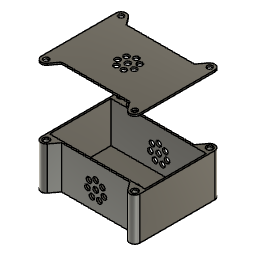
Boitier (Autodesk Fusion 360 design; units mm, degrees)
Autodesk Fusion 360 part; units mm, degrees
sketch "Esquisse2" plane through (0, 0, 0) normal (0, 0, 1) x (1, 0, 0)
  line L0 (29, -22) -> (29, 21.9996)
  line L1 (20, 19) -> (-20, 19)
  line L2 (-29, 21.9997) -> (-29, -21.9996)
  circle A0 centre (-26, -22) radius 1.4
  line L3 (-23.6, -23.8) -> (-20, -19)
  line L4 (-23.6, 23.8) -> (-20, 19)
  line L5 (23.6, -23.8) -> (20, -19)
  line L6 (23.6, 23.8) -> (20, 19)
  line L7 (-26.0004, -19) -> (-25.9996, -19)
  line L8 (-20, -19) -> (20, -19)
  arc A1 (-29, -21.9996) -> (-23.6, -23.8) centre (-26, -22) ccw
  circle A2 centre (-26, 22) radius 1.4
  circle A3 centre (26, 22) radius 1.4
  arc A4 (-23.6, 23.8) -> (-29, 21.9997) centre (-26, 22) ccw
  arc A5 (29, 21.9996) -> (23.6, 23.8) centre (26, 22) ccw
  arc A6 (23.6, -23.8) -> (29, -22) centre (26, -22) ccw
  line L9 (-28, -18) -> (28, -18)
  line L10 (28, -18) -> (28, 18)
  line L11 (28, 18) -> (-28, 18)
  line L12 (-28, 18) -> (-28, -18)
  circle A7 centre (26, -22) radius 1.4
  circle A8 centre (-26, -22) radius 1.55
  circle A9 centre (-26, 22) radius 1.55
  circle A10 centre (26, 22) radius 1.55
  circle A11 centre (26, -22) radius 1.55
  dimension "d16" = 2.8
  dimension "d17" = 2.8
  dimension "d19" = 2.8
  dimension "d20" = 2.8
  dimension "d21" = 3.1
  dimension "d22" = 3.1
  dimension "d23" = 3.1
  dimension "d24" = 3.1
  constraint horizontal L7
  constraint vertical L0
  constraint horizontal L1
  constraint vertical L2
  constraint concentric A0 A1
  constraint tangent L1 A4
  constraint tangent L1 A5
  constraint tangent L3 A1
  constraint coincident L3.end L7
  constraint tangent L4 A4
  constraint tangent L5 A6
  constraint tangent L6 A5
  constraint coincident L7.end A1
  constraint collinear L7 L8
  constraint concentric A2 A4
  constraint concentric A3 A5
  constraint horizontal L9
  constraint vertical L10
  constraint horizontal L11
  constraint vertical L12
  constraint concentric A6 A7
  constraint concentric A0 A8
  constraint concentric A2 A9
  constraint concentric A5 A10
  constraint concentric A6 A11
  measures "d16" diameter of A2
  measures "d17" diameter of A3
  measures "d19" diameter of A7
  measures "d20" diameter of A0
  measures "d21" diameter of A8
  measures "d22" diameter of A9
  measures "d23" diameter of A10
  measures "d24" diameter of A11
extrude "Extrusion1" add sketch "Esquisse2" along normal blind 1 contours L9 L10 L11 L12 makes body 1
extrude "Extrusion2" add sketch "Esquisse2" along normal blind 25 contours L0 L1 L2 L3 L4 L5 L6 L8 A1 A4 A5 A6 | A8 | A9 | A10 | A11 bodies 1
chamfer "Chanfrein1" distance 0.5 angle 45 4 edges at (-27.3053, 22.5063, 25) (24.6947, 22.5063, 25) (24.6947, -21.4937, 25) (-27.3053, -21.4937, 25) on bodies 1
extrude "Extrusion3" add sketch "Esquisse2" along normal blind 1 separate body contours L0 L1 L2 L3 L4 L5 L6 L8 A1 A4 A5 A6 | L9 L10 L11 L12 makes body 2
move_body "Déplacer1" bodies 2 to x (1, 0, 0) y (0, 1, 0) z (0, 0, 1) at (0, 0, 65)
cylinder "CylindrePrimitive1" add diameter 3.2 height 48 placed x (1, 0, 0) y (0, 0, -1) z (0, 1, 0) at (-55, 0, 20) separate body makes body 3
move_body "Déplacer2" bodies 3 to x (1, 0, 0) y (0, 1, 0) z (0, 0, 1) at (55, -24, -15)
copy_body "Copier/Coller des corps1" bodies 3 makes body 4
move_body "Déplacer3" bodies 4 to x (1, 0, 0) y (0, 1, 0) z (0, 0, 1) at (0, 0, -5)
pattern_circular "Réseau C1" count 7 over 360 about axis through (0, 1.75, 0) along (0, 1, 0) of bodies 3 makes body 5 at (5.0263, 8, 1.9721) makes body 6 at (4.6757, 8, -2.7002) makes body 7 at (0.7643, -8, -5.2701) makes body 8 at (-3.6729, 8, -3.9576) makes body 9 at (-5.308, -8, 0.4276) makes body 10 at (-3.0411, 8, 4.4615)
move_body "Déplacer4" bodies 10 9 8 7 6 5 4 3 to x (1, 0, 0) y (0, 1, 0) z (0, 0, 1) at (0, 0, 11)
copy_body "Copier/Coller des corps2" bodies 10 9 8 7 6 5 4 3 makes body 11 makes body 12 makes body 13 makes body 14 makes body 15 makes body 16 makes body 17 makes body 18
move_body "Déplacer5" bodies 11 12 13 14 15 16 17 18 to x (1, 0, 0) y (0, 0, -1) z (0, 1, 0) at (0, -11.1174, 59.6174)
copy_body "Copier/Coller des corps3" bodies 13 14 15 16 18 11 12 17 makes body 19 makes body 20 makes body 21 makes body 22 makes body 23 makes body 24 makes body 25 makes body 26
move_body "Déplacer6" bodies 19 20 21 22 23 24 25 26 to x (1, 0, 0) y (0, 1, 0) z (0, 0, 1) at (0, 0, -55)
combine "Combiner1" operation cut target body 1 tool bodies 3 5 6 7 8 9 10 4 20 19 22 23 26 21 25 24
combine "Combiner2" operation cut target body 2 tool bodies 13 14 15 16 18 11 12 17
